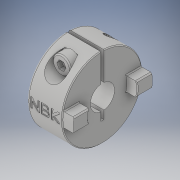
# Autodesk Inventor part: MOR-20C - 6-10 Hub 1
Saved by Autodesk Inventor 2019 (Build 230136000, 136)
## iProperties
Created: 2024-03-13
Part Number: MOR-20C - 6-10 Hub 1
Material: Generic
Catalog Web Link: www.cadenas.de
Description: MOR-C Hub 1-
Vendor: NBK
Document SubType Name: Modeling
Designer: psAdmin
Manufacturer: NBK
Mass: 2.46095 g
Surface Area: 16.1132 cm^2
Volume: 2.46095 cm^3
Density: 1 g/cm^3
Appearance: PSOLRGB-175-175-175
Category: PARTsolutions
Company: NBK
Title: MOR-20C - 6-10 Hub 1
Author: Cadenas PARTsolutions
PSOL_IDENT_0: {$CADENAS_DATA/23d-libs/nbk/motion_control_parts/couplicon_mini/oldham_type/mor/mor_c_1.prj},190 {VT
PSOL_IDENT_1: YP=3D},{NB=MOR-20C - 6-10 Hub 1},{LINA=MOR-20C - 6-10 Hub 1},{NN=MOR-C Hub 1},{DATE=12.03.2024 08:53
PSOL_IDENT_2: :06},{GEOMDATE=21.12.2021 07:12:10},{VERSION=},{LINEID=720},{WBVAR=D1D2},{WBNUMERIC=}  {NB=MOR-20C -
PSOL_IDENT_3: 6-10 Hub 1},{LINA=MOR-20C - 6-10 Hub 1},{KT=DUMMY},{CN=MOR-20C},{D1D2=6-10},{D1D2X1='5-5','5-6','5-
PSOL_IDENT_4: 6.35','5-8','5-9.525','5-10','6-6','6-6.35','6-8','6-9.525','6-10','6.35-6.35','6.35-8','6.35-9.525'
PSOL_IDENT_5: ,'6.35-10','8-8','8-9.525','8-10','9.525-9.525','9.525-10','10-10','1/4-1/4','1/4-5/16','1/4-3/8','5
PSOL_IDENT_6: /16-5/16','5/16-3/8','3/8-3/8','5-1/4','5-5/16','5-3/8','6-1/4','6-5/16','6-3/8','6.35-1/4','6.35-5/
PSOL_IDENT_7: 16','6.35-3/8','8-3/8','9.525-3/8','1/4-8','1/4-9.525','1/4-10','5/16-8','5/16-9.525','5/16-10','3/8
PSOL_IDENT_8: -10'},{A=20},{L=8.75},{W=27.4},{E=12.2},{F=4.38},{G=7.5},{M=M2.5},{D1=6},{D2=10},{NDM=2.50},{DV=10},
PSOL_IDENT_9: {DGV=4.5},{VGV=2.5},{SVD=1.1},{SV=2.0},{R3=5.0},{R2=3.0},{RZ=0.25},{DCT=0.8},{CT=15.00},{UV=3.30},{S
PSOL_IDENT_10: R=0.5},{SC=0.2},{KK=0.3},{KD=3.50},{KV=2.60}
NB: MOR-20C - 6-10 Hub 1
NN: MOR-C Hub 1
NBSYN: $CN. - $D1D2. Hub 1
LINA: MOR-20C - 6-10 Hub 1
CATALOG: NBK (Nabeya Bi-tech Kaisha
CN: MOR-20C
D1D2: 6-10
D1D2X1: '5-5','5-6','5-6.35','5-8','5-9.525','5-10','6-6','6-6.35','6-8','6-9.525','6-10','6.35-6.35','6.35-8','6.35-9.525','6.35-10','8-8','8-9.525','8-10','9.525-9.525','9.525-10','10-10','1/4-1/4','1/4-5/16','1/4-3/8','5/16-5/16','5/16-3/8','3/8-3/8','5-1/4','5-5/16','5-3/8','6-1/4','6-5/16','6-3/8','6.35-1/4','6.35-5/16','6.35-3/8','8-3/8','9.525-3/8','1/4-8','1/4-9.525','1/4-10','5/16-8','5/16-9.525','5/16-10','3/8-10'
A: 20
L: 8.75
W: 27.4
E: 12.2
F: 4.38
G: 7.5
M: M2.5
NDM: 2.5
DV: 10
DGV: 4.5
VGV: 2.5
SVD: 1.1
SV: 2
R3: 5
R2: 3
RZ: 0.25
DCT: 0.8
CT: 15
UV: 3.3
SR: 0.5
SC: 0.2
KK: 0.3
KD: 3.5
KV: 2.6
SUPPLIER: NBK
ARTICLENO: MOR-20C - 6-10 Hub 1
BOMINFO: MOR-20C - 6-10 Hub 1
CREATOR: CADENAS GmbH
Autodesk Inventor part; units mm, degrees
sketch "Sketch_1" plane through (0, 0, 0) normal (0, 0, 1) x (1, 0, 0)
  line L0 (11.35, 0) -> (0, 0)
  line L1 (0, 3.2) -> (0.2, 3)
  line L2 (0.2, 3) -> (8.75, 3)
  line L3 (8.75, 3) -> (8.75, 6.1)
  line L4 (8.75, 6.1) -> (11.15, 6.1)
  line L5 (11.15, 6.1) -> (11.35, 6.3)
  line L6 (11.35, 6.3) -> (11.35, 9.8)
  line L7 (11.35, 9.8) -> (8.75, 9.8)
  line L8 (8.75, 9.8) -> (8.55, 10)
  line L9 (8.55, 10) -> (0.5, 10)
  arc A0 (0.5, 10) -> (0, 9.5) centre (0.5, 9.5) ccw
  line L10 (0, 9.5) -> (0, 3.2)
  constraints: 22 end point, 2 point on circle, 1 centre point
revolve "Revolution1" add sketch "Sketch_1" angle 360 about axis through (11.35, 0, 0) along (1, 0, 0)
sketch "Sketch_2" plane through (0, 0, 0) normal (0, 0, 1) x (1, 0, 0)
  arc A0 (8.75, 2) -> (9, 1.75) centre (9, 2) ccw
  line L0 (9, 1.75) -> (11.05, 1.75)
  line L1 (11.05, 1.75) -> (11.35, 1.45)
  line L2 (11.35, 1.45) -> (11.35, -1.45)
  line L3 (11.35, -1.45) -> (11.05, -1.75)
  line L4 (11.05, -1.75) -> (9, -1.75)
  arc A1 (9, -1.75) -> (8.75, -2) centre (9, -2) ccw
  line L5 (8.75, -2) -> (8.75, -10)
  line L6 (8.75, -10) -> (12.35, -10)
  line L7 (12.35, -10) -> (12.35, 10)
  line L8 (12.35, 10) -> (8.75, 10)
  line L9 (8.75, 10) -> (8.75, 2)
  constraints: 20 end point, 4 point on circle, 2 centre point
extrude "Extrusion1" cut sketch "Sketch_2" along normal mid plane 20
sketch "Sketch_3" plane through (0, 7.5, 0) normal (0, 1, 0) x (1, 0, 0)
  line L0 (4.38, -10) -> (4.38, 10)
  line L1 (4.38, 10) -> (5.63, 10)
  line L2 (5.63, 10) -> (5.63, 0)
  line L3 (5.63, 0) -> (5.88, 0)
  line L4 (5.88, 0) -> (5.88, -3.3)
  line L5 (5.88, -3.3) -> (6.88, -3.3)
  line L6 (6.88, -3.3) -> (6.88, -10)
  line L7 (6.88, -10) -> (4.38, -10)
  line L8 (4.38, -10) -> (4.38, 10)
  constraints: 18 end point
revolve "Revolution2" cut sketch "Sketch_3" angle 360 about axis through (4.38, 7.5, 10) along (0, 0, 1)
sketch "Sketch_4" plane through (0, 0, 0) normal (1, 0, 0) x (0, 1, 0)
  line L0 (-5, 0.4) -> (-5, -0.4)
  line L1 (-5, -0.4) -> (10, -0.4)
  line L2 (10, -0.4) -> (10, 0.4)
  line L3 (10, 0.4) -> (-5, 0.4)
  constraints: 8 end point
extrude "Extrusion2" cut sketch "Sketch_4" along normal blind 8.75
sketch "Sketch_5" plane through (0, 7.5, 0) normal (0, 1, 0) x (1, 0, 0)
  line L0 (4.38, -5.8) -> (4.38, 4.2)
  line L1 (4.38, 4.2) -> (5.354, 4.2)
  line L2 (5.354, 4.2) -> (5.63, 3.924)
  line L3 (5.63, 3.924) -> (5.63, -3.3)
  line L4 (5.63, -3.3) -> (6.63, -3.3)
  line L5 (6.63, -3.3) -> (6.63, -5.5231)
  line L6 (6.63, -5.5231) -> (6.3531, -5.8)
  line L7 (6.3531, -5.8) -> (4.38, -5.8)
  line L8 (4.38, -5.8) -> (4.38, 4.2)
  constraints: 18 end point
revolve "Revolution3" add sketch "Sketch_5" angle 360 about axis through (4.38, 7.5, 5.8) along (0, 0, 1)
thread "Thread1" size "M2.5x0.45" class "6g" standard "ISO Metric profile" full length
sketch "Sketch_6" plane through (0, 0, 5.8) normal (0, 0, 1) x (1, 0, 0)
  line L0 (3.2253, 7.5) -> (3.8026, 6.5)
  line L1 (3.8026, 6.5) -> (4.9574, 6.5)
  line L2 (4.9574, 6.5) -> (5.5347, 7.5)
  line L3 (5.5347, 7.5) -> (4.9574, 8.5)
  line L4 (4.9574, 8.5) -> (3.8026, 8.5)
  line L5 (3.8026, 8.5) -> (3.2253, 7.5)
  constraints: 12 end point
extrude "Extrusion3" cut sketch "Sketch_6" against normal blind 1.1
sketch "Sketch_11" plane through (0, 0, 10) normal (0, 0, 1) x (1, 0, 0)
  line L0 (0.876, -1.2264) -> (1.314, -1.2264)
  line L1 (1.314, -1.2264) -> (1.314, 0.3504)
  line L2 (1.314, 0.3504) -> (2.5407, -1.0742)
  arc A0 (2.5407, -1.0742) -> (2.8726, -1.2264) centre (2.8726, -0.7884) ccw
  line L3 (2.8726, -1.2264) -> (3.1098, -1.2264)
  line L4 (3.1098, -1.2264) -> (3.1098, 1.2264)
  line L5 (3.1098, 1.2264) -> (2.6718, 1.2264)
  line L6 (2.6718, 1.2264) -> (2.6718, -0.3504)
  line L7 (2.6718, -0.3504) -> (1.4451, 1.0742)
  arc A1 (1.4451, 1.0742) -> (1.1132, 1.2264) centre (1.1132, 0.7884) ccw
  line L8 (1.1132, 1.2264) -> (0.876, 1.2264)
  line L9 (0.876, 1.2264) -> (0.876, -1.2264)
  constraints: 20 end point, 4 point on circle, 2 centre point
extrude "Extrusion4" cut sketch "Sketch_11" against normal blind 0.2
sketch "Sketch_12" plane through (0, 0, 10) normal (0, 0, 1) x (1, 0, 0)
  line L0 (3.504, -1.2264) -> (4.9494, -1.2264)
  arc A0 (4.9494, -1.2264) -> (5.2808, 0.0919) centre (4.9494, -0.5256) ccw
  arc A1 (5.2808, 0.0919) -> (4.7304, 1.2264) centre (4.7304, 0.5256) ccw
  line L1 (4.7304, 1.2264) -> (3.504, 1.2264)
  line L2 (3.504, 1.2264) -> (3.504, -1.2264)
  line L3 (3.8544, 0.1752) -> (4.7304, 0.1752)
  arc A2 (4.7304, 0.1752) -> (4.7304, 0.876) centre (4.7304, 0.5256) ccw
  line L4 (4.7304, 0.876) -> (3.8544, 0.876)
  line L5 (3.8544, 0.876) -> (3.8544, 0.1752)
  line L6 (3.8544, -0.876) -> (4.9494, -0.876)
  arc A3 (4.9494, -0.876) -> (4.9494, -0.1752) centre (4.9494, -0.5256) ccw
  line L7 (4.9494, -0.1752) -> (3.8544, -0.1752)
  line L8 (3.8544, -0.1752) -> (3.8544, -0.876)
  constraints: 18 end point, 8 point on circle, 4 centre point
extrude "Extrusion5" cut sketch "Sketch_12" against normal blind 0.2
sketch "Sketch_13" plane through (0, 0, 10) normal (0, 0, 1) x (1, 0, 0)
  line L0 (6.0006, -1.2264) -> (6.4386, -1.2264)
  line L1 (6.4386, -1.2264) -> (6.4386, -0.3407)
  line L2 (6.4386, -0.3407) -> (7.4588, -1.1341)
  arc A0 (7.4588, -1.1341) -> (7.7277, -1.2264) centre (7.7277, -0.7884) ccw
  line L3 (7.7277, -1.2264) -> (8.0154, -1.2264)
  line L4 (8.0154, -1.2264) -> (8.0154, -0.876)
  line L5 (8.0154, -0.876) -> (6.8891, 0)
  line L6 (6.8891, 0) -> (8.0154, 0.876)
  line L7 (8.0154, 0.876) -> (8.0154, 1.2264)
  line L8 (8.0154, 1.2264) -> (7.7277, 1.2264)
  arc A1 (7.7277, 1.2264) -> (7.4588, 1.1341) centre (7.7277, 0.7884) ccw
  line L9 (7.4588, 1.1341) -> (6.4386, 0.3407)
  line L10 (6.4386, 0.3407) -> (6.4386, 1.2264)
  line L11 (6.4386, 1.2264) -> (6.0006, 1.2264)
  line L12 (6.0006, 1.2264) -> (6.0006, -1.2264)
  constraints: 26 end point, 4 point on circle, 2 centre point
extrude "Extrusion6" cut sketch "Sketch_13" against normal blind 0.2
ref_plane "p1_dummy_XY" through (0, 0, 0) normal (1, 0, 0) x (0, 0, -1)
ref_plane "p1_dummy_YZ" through (0, 0, 0) normal (0, 0, -1) x (0, 1, 0)
ref_plane "p1_dummy_ZX" through (0, 0, 0) normal (0, 1, 0) x (1, 0, 0)
ref_plane "p1_p2_XY" through (9, 0, 0) normal (-1, 0, 0) x (0, 0, -1)
ref_plane "p1_p2_YZ" through (9, 0, 0) normal (0, 0, -1) x (0, -1, 0)
ref_plane "p1_p2_ZX" through (9, 0, 0) normal (0, -1, 0) x (-1, 0, 0)
body "Solid1"
